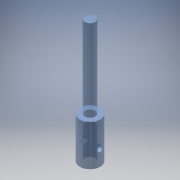
# Autodesk Inventor part: Part of Clutch
Saved by Autodesk Inventor 2016 (Build 200138000, 138)
## iProperties
Created: 2015-06-15
Part Number: Part of Clutch
Material: Aluminum 6061
Document SubType Name: Modeling
Designer: steele
Density: 2.7 g/cm^3
Appearance: Light Red
Author: steele
Autodesk Inventor part; units mm, degrees
ref_plane "XZ Plane" through (0, 0, 0) normal (0, 1, 0) x (-1, 0, 0)
ref_plane "XY Plane" through (0, 0, 0) normal (0, 0, 1) x (1, 0, 0)
sketch "Sketch1" plane through (0, 0, 0) normal (0, 1, 0) x (-1, 0, 0)
  circle A0 centre (0, 0) radius 12.7
  dimension "d0" = 25.4
  constraints: 1 centre point, 1 coincident
  measures "d0" diameter of A0
extrude "Extrusion1" add sketch "Sketch1" along normal blind 50.8
sketch "Sketch2" plane through (0, 50.8, 0) normal (0, 1, 0) x (1, 0, 0)
  circle A0 centre (0, 0) radius 6.35
  dimension "d3" = 12.7
  constraints: 1 centre point, 1 coincident
  measures "d3" diameter of A0
extrude "Extrusion2" add sketch "Sketch2" along normal blind 101.6
sketch "Sketch3" plane through (0, 0, 0) normal (0, -1, 0) x (1, 0, 0)
  circle A0 centre (0, 0) radius 6.35
  dimension "d6" = 12.7
  constraints: 1 centre point, 1 coincident
  measures "d6" diameter of A0
extrude "Extrusion3" cut sketch "Sketch3" against normal blind 38.1
ref_plane "Work Plane1" through (12.7, 0, 0) normal (1, 0, 0) x (0, 1, 0)
sketch "Sketch4" plane through (12.7, 0, 0) normal (1, 0, 0) x (0, 1, 0)
  line L0 (0, 0) -> (50.8, 0) construction
  line L1 (50.8, -12.7) -> (50.8, 12.7) construction
  line L2 (19.05, 12.7) -> (19.05, -12.7) construction
  line L3 (0, -12.7) -> (50.8, -12.7) construction
  line L4 (0, 12.7) -> (0, -12.7) construction
  circle A0 centre (19.05, 0) radius 3.302
  dimension "d10" = 19.05
  dimension "d11" = 6.604
  constraints: 4 end point, 2 midpoint, 1 centre point, 1 point on line, 1 vertical
  measures "d10" distance between parallel lines of L4 L2
  measures "d11" diameter of A0
extrude "Extrusion4" cut sketch "Sketch4" against normal through all
body "Solid1"
